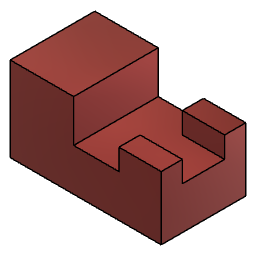
3d11 v1 (Autodesk Fusion 360 design; units mm, degrees)
Autodesk Fusion 360 part; units mm, degrees
sketch "Sketch1" plane through (0, 0, 0) normal (0, 0, 1) x (1, 0, 0)
  line L0 (0, 0) -> (0, 28)
  line L1 (0, 28) -> (21, 28)
  line L2 (21, 28) -> (21, 14)
  line L3 (21, 14) -> (36, 14)
  line L4 (36, 14) -> (36, 21)
  line L5 (36, 21) -> (50, 21)
  line L6 (50, 21) -> (50, 0)
  line L7 (50, 0) -> (0, 0)
  dimension "d1" = 21
  dimension "d2" = 14
  dimension "d3" = 14
  dimension "d4" = 21
  dimension "d5" = 28
  dimension "d6" = 7
  dimension "d7" = 50
  constraint coincident L0.start L7.end
  constraint vertical L0
  constraint perpendicular L0 L1
  constraint perpendicular L1 L2
  constraint perpendicular L2 L3
  constraint perpendicular L3 L4
  constraint perpendicular L4 L5
  constraint perpendicular L3 L6
  constraint perpendicular L0 L7
  measures "d1" distance of L0.end L1.end
  measures "d2" distance of L3 L7
  measures "d3" distance of L4.end L5.end
  measures "d4" distance of L5.end L6.end
  measures "d5" distance of L0.start L0.end
  measures "d6" distance of L3.end L4.end
  measures "d7" distance of L6.end L0.start
extrude "Extrude1" add sketch "Sketch1" along normal mid plane 28
sketch "Sketch2" plane through (0, 21, 0) normal (0, 1, 0) x (-1, 0, 0)
  line L0 (-36, -14) -> (-36, 14)
  line L1 (-36, 14) -> (-50, 14)
  line L2 (-50, 14) -> (-50, -14)
  line L3 (-50, -14) -> (-36, -14)
  line L4 (-36, -7) -> (-50, -7)
  line L5 (-36, 7) -> (-50, 7)
  dimension "d10" = 7
  dimension "d11" = 7
  constraint coincident L0 L4.start
  constraint coincident L2 L4.end
  constraint perpendicular L2 L4
  constraint coincident L0 L5.start
  constraint coincident L2 L5.end
  constraint perpendicular L2 L5
  measures "d10" distance of L3 L4
  measures "d11" distance of L1 L5
extrude "Extrude2" cut sketch "Sketch2" against normal up to surface (7 mm away) contours L0 L2 L4 L5
